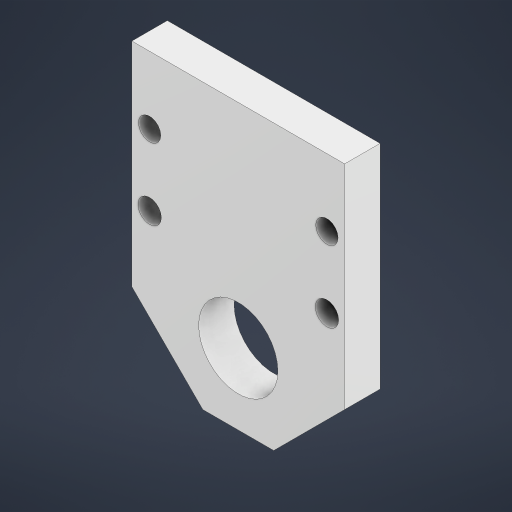
# Autodesk Inventor part: Lateral_Support_Connection2
Saved by Autodesk Inventor 2023 (Build 270158000, 158)
## iProperties
Created: 2023-11-22
Part Number: Lateral_Support_Connection2
Material: Polystyrene
Document SubType Name: Modeling
Designer: kelle
Density: 1.021 g/cm^3
Appearance: Smooth - White
Author: kelle
Autodesk Inventor part; units mm, degrees
ref_plane "YZ Plane" through (0, 0, 0) normal (1, 0, 0) x (0, 1, 0)
ref_plane "XZ Plane" through (0, 0, 0) normal (0, 1, 0) x (-1, 0, 0)
ref_plane "XY Plane" through (0, 0, 0) normal (0, 0, 1) x (1, 0, 0)
sketch "Sketch1" plane through (0, 0, 0) normal (0, 0, 1) x (1, 0, 0)
  line L0 (19.05, -25.4) -> (-19.05, -25.4)
  line L1 (-19.05, -25.4) -> (-19.05, 25.4)
  line L2 (-19.05, 25.4) -> (19.05, 25.4)
  line L3 (19.05, 25.4) -> (19.05, -25.4)
  line L4 (19.05, -25.4) -> (-19.05, 25.4) construction
  line L5 (-19.05, -25.4) -> (19.05, 25.4) construction
  point P0 (0, 0)
  dimension "d0" = 38.1
  dimension "d1" = 50.8
  constraints: 12 end point, 2 midpoint, 2 parallel, 1 horizontal, 1 perpendicular
  measures "d0" distance of L1.end L2.end
  measures "d1" distance of L0.end L1.end
extrude "Extrusion1" add sketch "Sketch1" along normal blind 6.35
chamfer "Chamfer1" distance 12.7 angle 45 2 edges at (19.05, -25.4, 3.175) (-19.05, -25.4, 3.175)
sketch "Sketch2" plane through (0, 0, 6.35) normal (0, 0, 1) x (1, 0, 0)
  line L0 (-19.05, 25.4) -> (-19.05, -12.7) construction
  line L1 (19.05, -12.7) -> (19.05, 25.4) construction
  line L2 (-19.05, -12.7) -> (19.05, -12.7) construction
  line L3 (-6.35, -25.4) -> (6.35, -25.4) construction
  line L4 (0, -25.4) -> (0, 0) construction
  circle A0 centre (0, -12.7) radius 7.1
  circle A1 centre (0, -12.7) radius 17.5 construction
  circle A2 centre (-15.875, 0.635) radius 2.1
  circle A3 centre (-15.875, 13.335) radius 2
  circle A4 centre (15.875, 0.635) radius 2.1
  circle A5 centre (15.875, 13.335) radius 2
  dimension "d7" = 14.2
  dimension "d8" = 12.7
  dimension "d9" = 35
  dimension "d10" = 4.2
  dimension "d11" = 13.335
  dimension "d12" = 3.175
  dimension "d13" = 4
  dimension "d14" = 12.7
  dimension "d15" = 3.175
  constraints: 6 centre point, 4 end point, 2 midpoint, 2 symmetric about line, 1 coincident, 1 horizontal, 1 parallel, 1 vertical, 2 other
  measures "d7" diameter of A0
  measures "d8" distance from line of L3 A0.centre
  measures "d9" diameter of A1
  measures "d10" diameter of A2
  measures "d11" distance from line of L2 A2.centre
  measures "d12" distance from line of L0 A2.centre
  measures "d13" diameter of A3
  measures "d14" distance of A2.centre A3.centre
  measures "d15" distance from line of L0 A3.centre
extrude "Extrusion2" cut sketch "Sketch2" against normal through all
body "Solid1"
